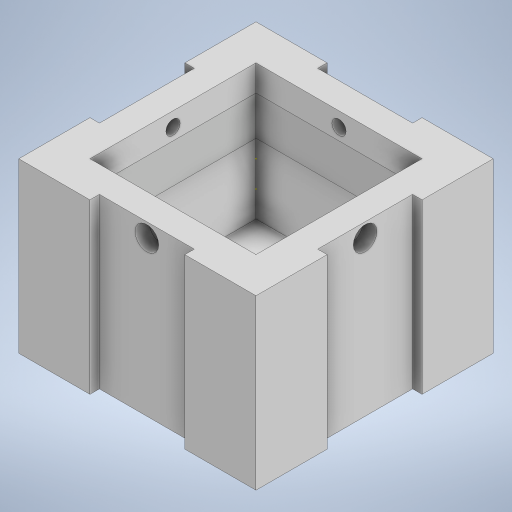
# Autodesk Inventor part: testpart
Saved by Autodesk Inventor 2023.1 (Build 271208000, 208)
## iProperties
Created: 2023-11-08
Part Number: testpart
Material: Generic
Document SubType Name: Modeling
Designer: Piotrek
Density: 1 g/cm^3
Appearance: Default
Author: Piotrek
Autodesk Inventor part; units mm, degrees
ref_plane "YZ Plane" through (0, 0, 0) normal (1, 0, 0) x (0, 1, 0)
ref_plane "XZ Plane" through (0, 0, 0) normal (0, 1, 0) x (-1, 0, 0)
ref_plane "XY Plane" through (0, 0, 0) normal (0, 0, 1) x (1, 0, 0)
sketch "Sketch1" plane through (0, 0, 0) normal (0, 1, 0) x (-1, 0, 0)
  line L0 (25, 25) -> (-25, 25)
  line L1 (-25, 25) -> (-25, -25)
  line L2 (-25, -25) -> (25, -25)
  line L3 (25, -25) -> (25, 25)
  line L4 (25, 25) -> (-25, -25) construction
  line L5 (-25, 25) -> (25, -25) construction
  line L6 (-22.5, 22.5) -> (22.5, 22.5)
  line L7 (22.5, 22.5) -> (22.5, -22.5)
  line L8 (22.5, -22.5) -> (-22.5, -22.5)
  line L9 (-22.5, -22.5) -> (-22.5, 22.5)
  line L10 (-22.5, 22.5) -> (22.5, -22.5) construction
  line L11 (22.5, 22.5) -> (-22.5, -22.5) construction
  point P0 (0, 0)
  dimension "d0" = 50
  dimension "d1" = 50
  dimension "d2" = 45
  dimension "d3" = 45
  constraints: 24 end point, 4 midpoint, 4 parallel, 2 horizontal, 2 perpendicular
  measures "d0" distance of L2.end L1.end
  measures "d1" distance of L1.end L0.end
  measures "d2" distance of L7.end L8.end
  measures "d3" distance of L6.end L7.end
extrude "Extrusion1" add sketch "Sketch1" along normal blind 30
extrude "Extrusion2" add sketch "Sketch1" along normal blind 2 contours L6 L7 L8 L9
sketch "Sketch2" plane through (0, 30, 0) normal (0, 1, 0) x (1, 0, 0)
  point P0 (0, 0)
sketch "Sketch3" plane through (0, 30, 0) normal (0, 1, 0) x (1, 0, 0)
  line L0 (17.5, -17.5) -> (-17.5, -17.5)
  line L1 (-17.5, -17.5) -> (-17.5, 17.5)
  line L2 (-17.5, 17.5) -> (17.5, 17.5)
  line L3 (17.5, 17.5) -> (17.5, -17.5)
  line L4 (17.5, -17.5) -> (-17.5, 17.5) construction
  line L5 (-17.5, -17.5) -> (17.5, 17.5) construction
  line L6 (-25, 25) -> (-25, -25) projected
  line L7 (25, -25) -> (-25, -25)
  line L8 (-25, -25) -> (-25, 25)
  line L9 (-25, 25) -> (25, 25)
  line L10 (25, 25) -> (25, -25)
  line L11 (25, -25) -> (-25, 25) construction
  line L12 (-25, -25) -> (25, 25) construction
  point P0 (0, 0)
  dimension "d8" = 35
  dimension "d9" = 35
  constraints: 24 end point, 4 midpoint, 4 parallel, 2 horizontal, 2 perpendicular
  measures "d8" distance of L1.end L2.end
  measures "d9" distance of L0.end L1.end
extrude "Extrusion3" add sketch "Sketch3" along normal blind 5.5
ref_plane "Work Plane1" through (0, 17.75, 0) normal (0, 1, 0) x (1, 0, 0)
chamfer "Chamfer1" distance 5 distance2 13.25 4 edges at (22.5, 30, 0) (0, 30, -22.5) (-22.5, 30, 0) (0, 30, 22.5) measured on face at (0, 30, 22) measured on face at (0, 30, -22) measured on face at (22, 30, 0) measured on face at (-22, 30, 0)
sketch "Sketch5" plane through (0, 35.5, 0) normal (0, 1, 0) x (1, 0, 0)
  point P0 (0, 0)
sketch "Sketch6" plane through (-17.5, 35.5, -17.5) normal (0, 0, 1) x (1, 0, 0)
  circle A0 centre (17.5, -3) radius 1.5
  line L0 (0, 0) -> (35, 0) projected
  point P0 (17.5, -35.5)
  point P1 (17.5, 0)
  dimension "d21" = 3
  dimension "d30" = 3
  constraints: 1 centre point, 1 midpoint
  measures "d21" diameter of A0
  measures "d30" distance of A0.centre point (17.5, 0)
extrude "Extrusion5" cut sketch "Sketch6" against normal through all
sketch "Sketch7" plane through (0, 35.5, 0) normal (0, 1, 0) x (1, 0, 0)
  line L0 (25, 25) -> (-25, 25) projected
  line L1 (10, 25) -> (0, 25)
  line L2 (10, 25) -> (-10, 25)
  line L3 (-10, 25) -> (10, 25)
  line L4 (10, 25) -> (10, 23)
  line L5 (10, 23) -> (-10, 23)
  line L6 (-10, 23) -> (-10, 25)
  point P0 (0, 0)
  dimension "d24" = 20
  dimension "d25" = 2
  constraints: 12 end point, 2 parallel, 2 point on line, 1 horizontal, 1 midpoint, 1 perpendicular
  measures "d24" distance of L1.start L2.end
  measures "d25" distance of L3.end L4.end
extrude "Extrusion6" cut sketch "Sketch7" against normal through all
sketch "Sketch9" plane through (10, 35.5, -23) normal (0, 0, -1) x (-1, 0, 0)
  circle A0 centre (10, -3) radius 1.5 projected
  circle A1 centre (10, -3) radius 2.5
  point P0 (10, -35.5)
  constraints: 1 centre point, 1 coincident
extrude "Extrusion7" cut sketch "Sketch9" against normal blind 3
pattern_circular "Circular Pattern2" count 4 over 360 about axis through (0, -10, 0) along (0, 1, 0) of "Extrusion7", "Extrusion6", "Extrusion5"
body "Solid1"
